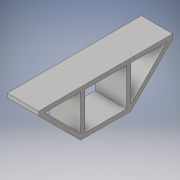
# Autodesk Inventor part: Motor_Shroud
Saved by Autodesk Inventor 2016 (Build 200138000, 138)
## iProperties
Created: 2018-10-20
Part Number: Motor_Shroud
Material: Generic
Document SubType Name: Modeling
Designer: Kyle
Density: 1 g/cm^3
Appearance: Default
Author: Kyle
Autodesk Inventor part; units mm, degrees
ref_plane "YZ Plane" through (0, 0, 0) normal (1, 0, 0) x (0, 1, 0)
ref_plane "XZ Plane" through (0, 0, 0) normal (0, 1, 0) x (-1, 0, 0)
ref_plane "XY Plane" through (0, 0, 0) normal (0, 0, 1) x (1, 0, 0)
sketch "Sketch1" plane through (0, 0, 0) normal (1, 0, 0) x (0, 1, 0)
  line L0 (9, 10) -> (-9, 10)
  line L1 (-9, 10) -> (-9, -10)
  line L2 (-9, -10) -> (9, -10)
  line L3 (9, -10) -> (9, 10)
  line L4 (9, 10) -> (-9, -10) construction
  line L5 (-9, 10) -> (9, -10) construction
  line L6 (-11, 12) -> (11, 12)
  line L7 (11, 12) -> (11, -12)
  line L8 (11, -12) -> (-11, -12)
  line L9 (-11, -12) -> (-11, 12)
  line L10 (-11, 12) -> (9, 32)
  line L11 (-11, 12) -> (21.2472, 12) construction
  line L12 (11, 12) -> (11, 32)
  line L13 (-11, -12) -> (9, -32)
  line L14 (-11, -12) -> (29.5291, -12) construction
  line L15 (11, -12) -> (11, -32)
  line L16 (9, 12) -> (9, 29.1716)
  line L17 (9, 29.1716) -> (-8.1716, 12)
  line L18 (-8.1716, -12) -> (9, -29.1716)
  line L19 (9, -29.1716) -> (9, -12)
  line L20 (11, 12) -> (11, 10)
  line L21 (11, 12) -> (9, 12)
  line L22 (-8.1716, 12) -> (-11, 12)
  line L23 (-11, -12) -> (-8.1716, -12)
  line L24 (11, -12) -> (9, -12)
  line L25 (9, 29.1716) -> (9, 32)
  line L26 (9, 32) -> (11, 32)
  line L27 (9, -29.1716) -> (11, -29.1716)
  line L28 (9, -29.1716) -> (9, -32)
  line L29 (9, -32) -> (11, -32)
  line L30 (11, 12) -> (9, 12)
  line L31 (-8.1716, 12) -> (-11, 12)
  line L32 (-8.1716, 12) -> (9, 29.1716)
  line L33 (-8.1716, -12) -> (9, -12)
  line L34 (11, -12) -> (9, -12)
  point P0 (0, 0)
  dimension "d0" = 18
  dimension "d1" = 20
  dimension "d2" = 2
  dimension "d3" = 45
  dimension "d4" = 45
  dimension "d5" = 2
  dimension "d6" = 2
  constraints: 70 end point, 7 collinear, 6 point on line, 5 parallel, 5 perpendicular, 4 horizontal, 3 vertical, 2 midpoint, 4 other
  measures "d0" distance of L2.end L1.end
  measures "d1" distance of L2.end L0.start
  measures "d2" distance between parallel lines of L0 L6
  measures "d3" angle of L11 L10
  measures "d4" angle of L13 L14
  measures "d5" distance between parallel lines of L12 L16
  measures "d6" distance between parallel lines of L13 L18
extrude "Extrusion2" add sketch "Sketch1" along normal blind 15 contours L10 L25 L17 L6 | L6 L7 L8 L9 | L8 L18 L28 L13 | L26 L12 L6 L16 L25 | L28 L27 L15 L29 | L8 L15 L27 L19
body "Solid2"
